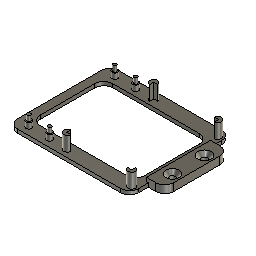
PicoHolder (Autodesk Fusion 360 design; units mm, degrees)
Autodesk Fusion 360 part; units mm, degrees
sketch "Sketch1" plane through (0, 0, 0) normal (0, 0, 1) x (1, 0, 0)
  line L0 (0, 0) -> (21, 0) construction
  line L1 (21, 0) -> (21, 51) construction
  line L2 (21, 51) -> (0, 51) construction
  line L3 (0, 51) -> (0, 0) construction
  line L4 (10.5, 51) -> (10.5, 0) construction
  line L5 (4.8, 51) -> (4.8, 0) construction
  line L6 (0, 49) -> (10.5, 49) construction
  circle A0 centre (4.8, 49) radius 1.05 construction
  line L7 (26, 49.05) -> (61, 49.05) construction
  line L8 (61, 49.05) -> (61, 1.95) construction
  line L9 (61, 1.95) -> (26, 1.95) construction
  line L10 (26, 1.95) -> (26, 49.05) construction
  line L11 (43.5, 49.05) -> (43.5, 1.95) construction
  line L12 (41.2, 1.95) -> (45.8, 1.95) construction
  line L13 (45.8, 1.95) -> (45.8, 0.45) construction
  line L14 (45.8, 0.45) -> (41.2, 0.45) construction
  line L15 (41.2, 0.45) -> (41.2, 1.95) construction
  line L16 (61, 27.8) -> (62.5, 27.8) construction
  line L17 (62.5, 27.8) -> (62.5, 23.2) construction
  line L18 (62.5, 23.2) -> (61, 23.2) construction
  line L19 (61, 23.2) -> (61, 27.8) construction
  line L20 (0, 25.5) -> (21, 25.5) construction
  line L21 (26, 25.5) -> (61, 25.5) construction
  circle A1 centre (43.5, 44.05) radius 1
  circle A2 centre (43.5, 6.95) radius 1
  line L22 (41.5, 49.05) -> (45.5, 49.05) construction
  line L23 (45.5, 49.05) -> (45.5, 47.55) construction
  line L24 (45.5, 47.55) -> (41.5, 47.55) construction
  line L25 (41.5, 47.55) -> (41.5, 49.05) construction
  line L26 (-2.0917, 53.1505) -> (64, 53.1505)
  line L27 (64, 53.1505) -> (64, -2.1505)
  line L28 (64, -2.1505) -> (-2.0917, -2.1505)
  line L29 (-2.0917, -2.1505) -> (-2.0917, 53.1505)
  circle A3 centre (4.8, 49) radius 1.55
  circle A4 centre (4.8, 49) radius 0.95
  line L30 (25.8, 49.25) -> (25.8, 47.06)
  line L31 (25.8, 49.25) -> (27.99, 49.25)
  arc A5 (27.99, 49.25) -> (25.8, 47.06) centre (26, 49.05) ccw
  line L32 (61.2, 49.25) -> (61.2, 47.06)
  line L33 (61.2, 49.25) -> (59.01, 49.25)
  arc A6 (61.2, 47.06) -> (59.01, 49.25) centre (61, 49.05) ccw
  line L34 (61.2, 1.75) -> (59.01, 1.75)
  line L35 (61.2, 1.75) -> (61.2, 3.94)
  arc A7 (59.01, 1.75) -> (61.2, 3.94) centre (61, 1.95) ccw
  line L36 (25.8, 1.75) -> (25.8, 3.94)
  line L37 (25.8, 1.75) -> (27.99, 1.75)
  arc A8 (25.8, 3.94) -> (27.99, 1.75) centre (26, 1.95) ccw
  circle A9 centre (16.2, 49) radius 0.95
  circle A10 centre (16.2, 49) radius 1.55
  circle A11 centre (4.8, 2) radius 0.95
  circle A12 centre (4.8, 2) radius 1.55
  circle A13 centre (16.2, 2) radius 0.95
  circle A14 centre (16.2, 2) radius 1.55
  dimension "d1" = 21
  dimension "d2" = 51
  dimension "d3" = 5.7
  dimension "d4" = 2
  dimension "d5" = 2.1
  dimension "d6" = 35
  dimension "d7" = 47.1
  dimension "d8" = 4.6
  dimension "d9" = 1.5
  dimension "d10" = 1.5
  dimension "d11" = 4.6
  dimension "d13" = 5
  dimension "d14" = 2
  dimension "d15" = 5
  dimension "d16" = 4
  dimension "d17" = 1.5
  dimension "d18" = 3
  dimension "d19" = 3
  dimension "d20" = 3
  dimension "d21" = 0.5
  dimension "d22" = -0.1
  dimension "d23" = 4
  dimension "d24" = 0.2
  dimension "d25" = 0.2
  constraint horizontal L0
  constraint vertical L1
  constraint horizontal L2
  constraint vertical L3
  constraint coincident L0.start L3.end
  constraint midpoint L2 L4.start
  constraint midpoint L0 L4.end
  constraint coincident L2 L5.start
  constraint coincident L0 L5.end
  constraint perpendicular L0 L5
  constraint coincident L3 L6.start
  constraint coincident L4 L6.end
  constraint perpendicular L4 L6
  constraint coincident L6 A0.centre
  constraint coincident L5 A0.centre
  constraint horizontal L7
  constraint vertical L8
  constraint horizontal L9
  constraint vertical L10
  constraint midpoint L7 L11.start
  constraint midpoint L9 L11.end
  constraint horizontal L12
  constraint vertical L13
  constraint horizontal L14
  constraint vertical L15
  constraint midpoint L9 L12
  constraint horizontal L16
  constraint vertical L17
  constraint horizontal L18
  constraint vertical L19
  constraint midpoint L8 L19
  constraint midpoint L3 L20.start
  constraint midpoint L1 L20.end
  constraint midpoint L10 L21.start
  constraint midpoint L8 L21.end
  constraint horizontal L20.end L21.start
  constraint coincident L11 A1.centre
  constraint symmetric L21 A1 A2
  constraint horizontal L22
  constraint vertical L23
  constraint horizontal L24
  constraint vertical L25
  constraint midpoint L7 L22
  constraint horizontal L26
  constraint vertical L27
  constraint horizontal L28
  constraint vertical L29
  constraint coincident L7.start L10.end
  constraint perpendicular L7 L30
  constraint perpendicular L30 L31
  constraint symmetric L11 L30.start L32.start
  constraint symmetric L11 L30.end L32.end
  constraint symmetric L11 L31.end L33.end
  constraint symmetric L11 A5 A6
  constraint symmetric L21 L30.start L36.start
  constraint symmetric L21 L30.end L36.end
  constraint symmetric L21 L31.end L37.end
  constraint symmetric L21 A5 A8
  constraint symmetric L21 L32.start L34.start
  constraint symmetric L21 L32.end L35.end
  constraint symmetric L21 L33.end L34.end
  constraint symmetric L21 A6 A7
  constraint symmetric L4 A3 A10
  constraint symmetric L4 A4 A9
  constraint symmetric L20 A3 A12
  constraint symmetric L20 A4 A11
  constraint symmetric L20 A9 A13
  constraint symmetric L20 A10 A14
  measures "d1" distance of L0.start L0.end
  measures "d2" distance of L0.start L2.end
  measures "d3" distance of L4 L5
  measures "d4" distance of L2 L6
  measures "d5" diameter of A0
  measures "d6" distance of L7.start L7.end
  measures "d7" distance of L7.start L9.end
  measures "d8" distance of L12.start L12.end
  measures "d9" distance of L12.start L14.end
  measures "d10" distance of L16.start L16.end
  measures "d11" distance of L16.start L18.end
  measures "d13" distance of L1 L10
  measures "d14" diameter of A1
  measures "d15" distance of L11.start A1.centre
  measures "d16" distance of L22.start L22.end
  measures "d17" distance of L22.start L24.end
  measures "d18" distance of L2.end L26.start
  measures "d19" distance of L0.start L28.end
  measures "d20" distance of L8 L27
  measures "d23" diameter of A5
  measures "d24" distance of L10 L30
  measures "d25" distance of L7 L31
extrude "Extrude1" add sketch "Sketch1" along normal blind 2 contours L26 L27 L28 L29 makes body 1
extrude "Extrude2" add sketch "Sketch1" along normal blind 5 contours A3 | A10 | A12 | A14 bodies 1
extrude "Extrude3" add sketch "Sketch1" along normal blind 8 contours A4 | A9 | A11 | A13 bodies 1
extrude "Extrude4" add sketch "Sketch1" along normal blind 10 contours L30 L31 A5 | L32 L33 A6 | L34 L35 A7 | L36 L37 A8 bodies 1
fillet "Fillet1" radius 5 4 edges at (-2.0917, -2.1505, 1) (64, -2.1505, 1) (64, 53.1505, 1) (-2.0917, 53.1505, 1) on bodies 1
sketch "Sketch2" plane through (0, 0, 2) normal (0, 0, 1) x (-1, 0, 0)
  line L0 (-59.01, -1.75) -> (-61.2, -1.75)
  line L1 (-61.2, -1.75) -> (-61.2, -3.94)
  arc A0 (-59.01, -1.75) -> (-61.2, -3.94) centre (-61, -1.95) ccw
  circle A1 centre (-16.2, -49) radius 1.55
  line L2 (-61.2, -47.06) -> (-61.2, -49.25)
  line L3 (-61.2, -49.25) -> (-59.01, -49.25)
  arc A2 (-61.2, -47.06) -> (-59.01, -49.25) centre (-61, -49.05) ccw
  line L4 (-25.8, -3.94) -> (-25.8, -1.75)
  line L5 (-25.8, -1.75) -> (-27.99, -1.75)
  arc A3 (-25.8, -3.94) -> (-27.99, -1.75) centre (-26, -1.95) ccw
  circle A4 centre (-4.8, -2) radius 1.55
  circle A5 centre (-43.5, -44.05) radius 1
  circle A6 centre (-43.5, -6.95) radius 1
  circle A7 centre (-4.8, -49) radius 1.55
  line L6 (-27.99, -49.25) -> (-25.8, -49.25)
  line L7 (-25.8, -49.25) -> (-25.8, -47.06)
  arc A8 (-27.99, -49.25) -> (-25.8, -47.06) centre (-26, -49.05) ccw
  circle A9 centre (-16.2, -2) radius 1.55
  arc A10 (-2.9083, -53.1505) -> (2.0917, -48.1505) centre (-2.9083, -48.1505) ccw
  line L8 (2.0917, -48.1505) -> (2.0917, -2.8495)
  arc A11 (2.0917, -2.8495) -> (-2.9083, 2.1505) centre (-2.9083, -2.8495) ccw
  line L9 (-2.9083, 2.1505) -> (-59, 2.1505)
  arc A12 (-59, 2.1505) -> (-64, -2.8495) centre (-59, -2.8495) ccw
  line L10 (-64, -2.8495) -> (-64, -48.1505)
  arc A13 (-64, -48.1505) -> (-59, -53.1505) centre (-59, -48.1505) ccw
  line L11 (-59, -53.1505) -> (-2.9083, -53.1505)
  line L12 (2.0917, -53.1505) -> (-64, 2.1505) construction
  line L13 (2.0917, 2.1505) -> (-64, -53.1505) construction
  line L14 (-59.4991, -5.6547) -> (-2.4092, -5.6547)
  line L15 (-2.4092, -5.6547) -> (-2.4092, -45.3453)
  line L16 (-2.4092, -45.3453) -> (-59.4991, -45.3453)
  line L17 (-59.4991, -45.3453) -> (-59.4991, -5.6547)
  line L18 (-59.4991, -5.6547) -> (-2.4092, -45.3453) construction
  line L19 (-2.4092, -5.6547) -> (-59.4991, -45.3453) construction
  point P0 (2.0917, -53.1505)
  point P1 (-64, 2.1505)
  point P2 (2.0917, 2.1505)
  point P3 (-64, -53.1505)
  point P4 (-30.9541, -25.5)
  constraint coincident P0 L12.start
  constraint coincident P1 L12.end
  constraint coincident P2 L13.start
  constraint coincident P3 L13.end
  constraint horizontal L14
  constraint perpendicular L14 L15
  constraint parallel L14 L16
  constraint parallel L15 L17
  constraint coincident L18 P4
  constraint coincident L19 P4
  constraint midpoint L13 P4
extrude "Extrude5" cut sketch "Sketch2" against normal up to surface (2 mm away) contours L14 L15 L16 L17 bodies 1
fillet "Fillet2" radius 5 4 edges at (2.4092, 45.3453, 1) (59.4991, 45.3453, 1) (59.4991, 5.6547, 1) (2.4092, 5.6547, 1) on bodies 1
sketch "Sketch3" plane through (0, 0, 0) normal (0, 0, 1) x (1, 0, 0)
  line L0 (73, 43) -> (63, 43)
  line L1 (63, 43) -> (63, 8)
  line L2 (63, 8) -> (73, 8)
  line L3 (73, 8) -> (73, 43)
  line L4 (64, 43) -> (64, 8) construction
  line L5 (64, 53.1505) -> (64, -2.1505)
  line L6 (64, 43) -> (73, 25.5) construction
  line L7 (73, 25.5) -> (64, 8) construction
  circle A0 centre (68.5, 16.75) radius 1.6
  circle A1 centre (68.5, 34.25) radius 1.6
  dimension "d90" = 35
  dimension "d91" = 1
  dimension "d93" = 10
  dimension "d94" = 3.2
  dimension "d95" = 3.2
  constraint horizontal L0
  constraint vertical L1
  constraint horizontal L2
  constraint vertical L3
  constraint coincident L0 L4.start
  constraint perpendicular L0 L4
  constraint coincident L2 L4.end
  constraint midpoint L4 L5
  constraint midpoint L3 L6.end
  constraint midpoint L7 A0.centre
  constraint midpoint L6 A1.centre
  measures "d90" distance of L0.start L2.end
  measures "d91" distance of L1 L4
  measures "d93" distance of L1.end L2.end
  measures "d94" diameter of A0
  measures "d95" diameter of A1
extrude "Extrude6" add sketch "Sketch3" along normal blind 4.2 separate body contours L0 L2 L3 L5 makes body 2
extrude "Extrude7" add sketch "Sketch3" along normal blind 2 from surface at 2.2 contours L0 L1 L2 L5 bodies 1 2
chamfer "Chamfer1" distance 2 angle 45 2 edges at (67.0083, 17.3286, 4.2) (67.0083, 34.8286, 4.2) on bodies 2
fillet "Fillet3" radius 5 2 edges at (73, 8, 2.1) (73, 43, 2.1) on bodies 2
equation "d3 = ( 11.4 / 2 ) * 1 mm"
named bodies: "Holder", "ClipOn"
